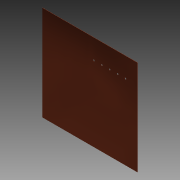
# Autodesk Inventor part: 2221B_Copper Box Side_Feedthrough_V1
Saved by Autodesk Inventor 2020 (Build 240168000, 168)
## iProperties
Created: 2017-08-01
Part Number: 2221B_Copper Box Side_Feedthrough_V1
Material: Copper
Document SubType Name: Modeling
Designer: MPI
Density: 8.94 g/cm^3
Appearance: Copper - Satin
Author: MPI
Autodesk Inventor part; units mm, degrees
ref_plane "YZ Plane" through (0, 0, 0) normal (1, 0, 0) x (0, 1, 0)
ref_plane "XZ Plane" through (0, 0, 0) normal (0, 1, 0) x (-1, 0, 0)
ref_plane "XY Plane" through (0, 0, 0) normal (0, 0, 1) x (1, 0, 0)
sketch "Sketch1" plane through (0, 0, 0) normal (0, 0, 1) x (1, 0, 0)
  line L0 (-304.8, -304.8) -> (304.8, -304.8)
  line L1 (304.8, -304.8) -> (304.8, 304.8)
  line L2 (304.8, 304.8) -> (-304.8, 304.8)
  line L3 (-304.8, 304.8) -> (-304.8, -304.8)
  line L4 (-304.8, -304.8) -> (304.8, 304.8) construction
  line L5 (304.8, -304.8) -> (-304.8, 304.8) construction
  point P0 (0, 0)
  dimension "d0" = 609.6
  dimension "d1" = 609.6
  constraints: 12 end point, 2 midpoint, 2 parallel, 1 horizontal, 1 perpendicular
  measures "d0" distance of L2.end L1.end
  measures "d1" distance of L1.end L0.end
extrude "Extrusion1" add sketch "Sketch1" along normal blind 1.0668
sketch "Sketch2" plane through (0, 0, 0) normal (0, 0, -1) x (-1, 0, 0)
  line L0 (304.8, -304.8) -> (-304.8, -304.8) projected
  line L1 (304.8, 304.8) -> (304.8, -304.8) projected
  line L2 (-304.8, 304.8) -> (304.8, 304.8) projected
  line L3 (-304.8, -304.8) -> (-304.8, 304.8) projected
  line L4 (-304.8, -304.8) -> (-304.8, 304.8) projected
  line L5 (-304.8, 177.8) -> (304.8, 177.8) construction
  line L6 (304.8, 304.8) -> (304.8, -304.8) projected
  circle A0 centre (-228.6, 177.8) radius 5
  circle A1 centre (-177.8, 177.8) radius 5
  circle A2 centre (-127, 177.8) radius 5
  circle A3 centre (-76.2, 177.8) radius 5
  circle A4 centre (-25.4, 177.8) radius 5
  point P0 (0, 0)
  dimension "d4" = 127
  dimension "d5" = 10
  dimension "d6" = 76.2
  dimension "d9" = 50.8
  constraints: 5 centre point, 3 point on line, 2 end point, 1 horizontal, 1 perpendicular, 8 other
  measures "d4" distance between parallel lines of L2 L5
  measures "d5" diameter of A0
  measures "d6" distance from line of L3 A0.centre
  measures "d9" distance of A0.centre A1.centre
extrude "Extrusion2" cut sketch "Sketch2" against normal through all contours A0 | A1 | A2 | A3 | A4
body "Solid1"
